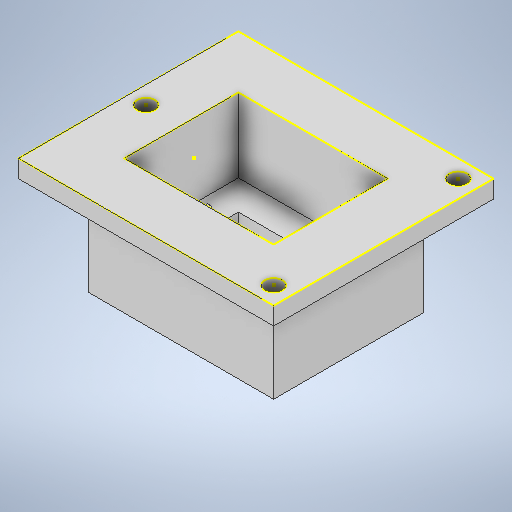
# Autodesk Inventor part: servo_holder_V2
Saved by Autodesk Inventor 2025.3 (Build 293356000, 356)
## iProperties
Created: 2026-04-11
Part Number: servo_holder_V2
Material: Generic
Document SubType Name: Modeling
Designer: kamal
Density: 1 g/cm^3
Appearance: Default
Author: kamal
## iProperties of the stored document servo_holder_V2_3DPrint.ipt
Created: 2026-04-12
Part Number: servo_holder_V2_3DPrint
Material: Generic
Document SubType Name: Modeling
Designer: kamal
Density: 1 g/cm^3
Appearance: Default
Author: kamal
Autodesk Inventor part; units mm, degrees
ref_plane "YZ Plane" through (0, 0, 0) normal (1, 0, 0) x (0, 1, 0)
ref_plane "XZ Plane" through (0, 0, 0) normal (0, 1, 0) x (-1, 0, 0)
sketch "Sketch1" plane through (0, 0, 0) normal (0, 0, 1) x (1, 0, 0)
  line L0 (0, 0) -> (22.6, 0)
  line L1 (22.6, 0) -> (22.6, 12.6)
  line L2 (22.6, 12.6) -> (0, 12.6)
  line L3 (0, 12.6) -> (0, 0)
  line L4 (-4.9, 17.5) -> (27.5, 17.5)
  line L5 (27.5, 17.5) -> (27.5, -4.9)
  line L6 (27.5, -4.9) -> (-4.9, -4.9)
  line L7 (-4.9, -4.9) -> (-4.9, 17.5)
  dimension "d0" = 22.6
  dimension "d1" = 12.6
  dimension "d2" = 4.9
  constraints: 16 end point, 4 parallel, 2 perpendicular, 1 horizontal, 3 other
  measures "d0" distance of L2.end L1.end
  measures "d1" distance of L1.end L0.end
  measures "d2" distance between parallel lines of L2 L4
extrude "Extrusion1" add sketch "Sketch1" along normal blind 17
sketch "Sketch2" plane through (0, 0, 0) normal (0, 0, -1) x (-1, 0, 0)
  line L0 (4.9, -4.9) -> (-27.5, -4.9) projected
  line L1 (-27.5, -4.9) -> (-27.5, 17.5) projected
  line L2 (-27.5, 17.5) -> (4.9, 17.5) projected
  line L3 (4.9, 17.5) -> (4.9, -4.9) projected
  point P0 (0, 0)
extrude "Extrusion2" add sketch "Sketch2" along normal blind 5
sketch "Sketch3" plane through (0, 0, 17) normal (0, 0, 1) x (1, 0, 0)
  line L0 (-4.9, -4.9) -> (27.5, -4.9) projected
  line L1 (27.5, -4.9) -> (27.5, 17.5) projected
  line L2 (27.5, 17.5) -> (-4.9, 17.5) projected
  line L3 (-4.9, 17.5) -> (-4.9, -4.9) projected
  line L4 (0, 0) -> (0, 12.6) projected
  line L5 (0, 12.6) -> (22.6, 12.6) projected
  line L6 (22.6, 12.6) -> (22.6, 0) projected
  line L7 (22.6, 0) -> (0, 0) projected
  line L8 (-9.9, -9.9) -> (32.5, -9.9)
  line L9 (32.5, -9.9) -> (32.5, 22.5)
  line L10 (32.5, 22.5) -> (-9.9, 22.5)
  line L11 (-9.9, 22.5) -> (-9.9, -9.9)
  line L12 (-4.9, 6.3) -> (-2.6, 6.3) construction
  line L13 (27.5, 17.5) -> (27.5, -4.9) projected
  line L14 (27.5, 6.3) -> (25.2, 6.3) construction
  circle A0 centre (-2.6, 6.3) radius 1
  circle A1 centre (25.2, 6.3) radius 1
  dimension "d7" = 5
  dimension "d10" = 2.3
  dimension "d11" = 2.3
  dimension "d12" = 2
  dimension "d13" = 2
  constraints: 12 end point, 2 centre point, 2 coincident, 2 horizontal, 2 midpoint, 3 other
  measures "d7" distance between parallel lines of L3 L11
  measures "d10" distance of L12.start L12.end
  measures "d11" distance of L14.start L14.end
  measures "d12" diameter of A0
  measures "d13" diameter of A1
extrude "Extrusion4" add sketch "Sketch3" along normal blind 5 contours A0 | A1
chamfer "Chamfer1" distance 0.5 angle 45 2 edges at (-3.6, 6.3, 22) (24.2, 6.3, 22)
ref_plane "Work Plane1" through (0, 0, 12) normal (0, 0, 1) x (1, 0, 0)
sketch "Sketch5" plane through (0, 0, 12) normal (0, 0, 1) x (1, 0, 0)
  line L0 (-4.9, -4.9) -> (27.5, -4.9) projected
  line L1 (27.5, -4.9) -> (27.5, 17.5) projected
  line L2 (27.5, 17.5) -> (-4.9, 17.5) projected
  line L3 (-4.9, 17.5) -> (-4.9, -4.9) projected
  line L4 (32.5, -9.9) -> (-9.9, -9.9)
  line L5 (-9.9, -9.9) -> (-9.9, 22.5)
  line L6 (-9.9, 22.5) -> (32.5, 22.5)
  line L7 (32.5, 22.5) -> (32.5, -9.9)
  point P0 (0, 0)
  dimension "d21" = 5
  constraints: 8 end point, 3 other
  measures "d21" distance between parallel lines of L0 L4
extrude "Extrusion5" add sketch "Sketch5" along normal blind 5
sketch "Sketch14" plane through (0, 0, 17) normal (0, 0, 1) x (1, 0, 0)
  line L0 (22.6, 12.6) -> (22.6, 0) projected
  line L1 (0, 12.6) -> (22.6, 12.6) projected
  line L2 (0, 0) -> (0, 12.6) projected
  line L3 (22.6, 0) -> (0, 0) projected
  line L4 (-9.9, -9.9) -> (-9.9, 22.5)
  line L5 (-9.9, 22.5) -> (32.5, 22.5)
  line L6 (32.5, 22.5) -> (32.5, -9.9)
  line L7 (32.5, -9.9) -> (-9.9, -9.9)
  line L8 (-14.9, -14.9) -> (-14.9, 27.5)
  line L9 (-14.9, 27.5) -> (37.5, 27.5)
  line L10 (37.5, 27.5) -> (37.5, -14.9)
  line L11 (37.5, -14.9) -> (-14.9, -14.9)
  dimension "d52" = 9.9
  dimension "d53" = 5
  constraints: 16 end point, 6 other
  measures "d52" distance between parallel lines of L3 L7
  measures "d53" distance between parallel lines of L7 L11
extrude "Extrusion11" add sketch "Sketch14" along normal blind 16 contours L8 L9 L10 L11
sketch "Sketch15" plane through (0, 0, 33) normal (0, 0, 1) x (1, 0, 0)
  line L0 (-14.9, 27.5) -> (-14.9, -14.9) projected
  line L1 (-14.9, -14.9) -> (37.5, -14.9) projected
  line L2 (37.5, -14.9) -> (37.5, 27.5) projected
  line L3 (37.5, 27.5) -> (-14.9, 27.5) projected
  line L4 (47.5, -24.9) -> (-24.9, -24.9)
  line L5 (-24.9, -24.9) -> (-24.9, 37.5)
  line L6 (-24.9, 37.5) -> (47.5, 37.5)
  line L7 (47.5, 37.5) -> (47.5, -24.9)
  line L8 (32.5, -9.9) -> (-9.9, -9.9) projected
  line L9 (-9.9, -9.9) -> (-9.9, 22.5) projected
  line L10 (-9.9, 22.5) -> (32.5, 22.5) projected
  line L11 (32.5, 22.5) -> (32.5, -9.9) projected
  point P0 (0, 0)
  dimension "d56" = 10
  constraints: 8 end point, 3 other
  measures "d56" distance between parallel lines of L1 L4
extrude "Extrusion12" add sketch "Sketch15" along normal blind 5 contours L3 L2 L1 L0 | L4 L5 L6 L7
sketch "Sketch16" plane through (0, 0, 33) normal (0, 0, -1) x (-1, 0, 0)
  line L0 (-37.5, -14.9) -> (-37.5, 27.5) projected
  line L1 (14.9, -14.9) -> (-37.5, -14.9) projected
  line L2 (14.9, 27.5) -> (14.9, -14.9) projected
  line L3 (-37.5, 27.5) -> (14.9, 27.5) projected
  line L4 (9.9, 22.5) -> (9.9, -9.9) projected
  line L5 (9.9, -9.9) -> (-32.5, -9.9) projected
  line L6 (-32.5, -9.9) -> (-32.5, 22.5) projected
  line L7 (-32.5, 22.5) -> (9.9, 22.5) projected
  line L8 (-42.5, 32.5) -> (-42.5, -19.9) construction
  line L9 (-42.5, -19.9) -> (19.9, -19.9) construction
  line L10 (19.9, -19.9) -> (19.9, 32.5) construction
  line L11 (19.9, 32.5) -> (-42.5, 32.5) construction
  circle A0 centre (19.9, 6.3) radius 2.5
  circle A1 centre (-42.5, 32.5) radius 2.5
  circle A2 centre (-42.5, -19.9) radius 2.5
  point P0 (0, 0)
  dimension "d59" = 5
  dimension "d60" = 5
  dimension "d61" = 5
  dimension "d62" = 5
  constraints: 8 end point, 3 centre point, 2 coincident, 1 midpoint, 3 other
  measures "d59" distance between parallel lines of L0 L8
  measures "d60" diameter of A0
  measures "d61" diameter of A1
  measures "d62" diameter of A2
extrude "Extrusion13" cut sketch "Sketch16" against normal blind 5 contours A0 | A1 | A2
sketch "Sketch17" plane through (-4.9, -4.9, -5) normal (-1, 0, 0) x (0, 0, 1)
  line L0 (-10, 15.2) -> (10, 15.2)
  line L1 (10, 15.2) -> (10, 7.2)
  line L2 (10, 7.2) -> (-10, 7.2)
  line L3 (-10, 7.2) -> (-10, 15.2)
  line L4 (0, 22.4) -> (0, 0) projected
  line L5 (-10, 15.2) -> (10, 7.2) construction
  line L6 (10, 15.2) -> (-10, 7.2) construction
  line L7 (5, 15.2) -> (5, 7.2)
  line L8 (0, 11.2) -> (5, 11.2)
  point P0 (5, 4.9)
  dimension "d65" = 20
  dimension "d66" = 8
  dimension "d67" = 5
  constraints: 16 end point, 4 midpoint, 2 parallel, 2 perpendicular, 2 point on line, 1 horizontal
  measures "d65" distance of L1.end L2.end
  measures "d66" distance of L0.end L1.end
  measures "d67" distance of L8.start L8.end
extrude "Extrusion14" cut sketch "Sketch17" against normal blind 5 contours L0 L1 L2 L7
sketch "Sketch18" plane through (0, 0, 12) normal (0, 0, -1) x (-1, 0, 0)
  line L0 (-32.5, 22.5) -> (9.9, 22.5) projected
  line L1 (-32.5, -9.9) -> (-32.5, 22.5) projected
  line L2 (9.9, -9.9) -> (-32.5, -9.9) projected
  line L3 (9.9, 22.5) -> (9.9, -9.9) projected
  line L4 (4.9, -4.9) -> (4.9, 17.5) projected
  line L5 (-27.5, -4.9) -> (4.9, -4.9) projected
  line L6 (-27.5, 17.5) -> (-27.5, -4.9) projected
  line L7 (4.9, 17.5) -> (-27.5, 17.5) projected
  point P0 (0, 0)
extrude "Extrusion15" add sketch "Sketch18" along normal blind 7
sketch "Sketch20" plane through (-4.9, -4.9, -5) normal (-1, 0, 0) x (0, 0, 1)
  line L0 (5, 7.2) -> (0, 7.2)
  line L1 (5, 15.2) -> (10, 15.2) projected
  line L2 (5, 15.2) -> (0, 15.2)
  line L3 (0, 15.2) -> (0, 7.2)
  line L4 (5, 15.2) -> (5, 17.5) projected
  line L5 (5, 7.2) -> (5, 15.2)
  point P0 (5, 4.9)
  dimension "d74" = 10
  constraints: 8 end point, 2 horizontal, 1 collinear, 1 perpendicular
  measures "d74" distance from line of L1.end L3
extrude "Extrusion17" cut sketch "Sketch20" against normal blind 12
sketch "Sketch21" plane through (0, 0, 17) normal (0, 0, -1) x (-1, 0, 0)
  line L0 (-32.5, -9.9) -> (9.9, -9.9) projected
  line L1 (9.9, -9.9) -> (9.9, 22.5) projected
  line L2 (9.9, 22.5) -> (-32.5, 22.5) projected
  line L3 (-32.5, 22.5) -> (-32.5, -9.9) projected
  line L4 (0, 2.3) -> (0, 10.3) projected
  line L5 (4.9, 2.3) -> (0, 2.3) projected
  line L6 (4.9, -4.9) -> (4.9, 2.3) projected
  line L7 (-27.5, -4.9) -> (4.9, -4.9) projected
  line L8 (-27.5, 17.5) -> (-27.5, -4.9) projected
  line L9 (4.9, 17.5) -> (-27.5, 17.5) projected
  line L10 (4.9, 10.3) -> (4.9, 17.5) projected
  line L11 (4.9, 10.3) -> (0, 10.3) projected
  line L12 (-37.5, -14.9) -> (-37.5, 27.5) projected
  line L13 (14.9, -14.9) -> (-37.5, -14.9) projected
  line L14 (14.9, 27.5) -> (14.9, -14.9) projected
  line L15 (-37.5, 27.5) -> (14.9, 27.5) projected
  line L16 (9.9, 22.5) -> (9.9, -9.9) projected
  line L17 (9.9, -9.9) -> (-32.5, -9.9) projected
  line L18 (-32.5, -9.9) -> (-32.5, 22.5) projected
  line L19 (-32.5, 22.5) -> (9.9, 22.5) projected
  point P0 (0, 0)
extrude "Extrusion18" add sketch "Sketch21" along normal blind 12 contours L12 L15 L14 L13
sketch "Sketch22" plane through (0, 0, 17) normal (0, 0, 1) x (1, 0, 0)
  line L0 (0, 12.6) -> (22.6, 12.6) projected
  line L1 (22.6, 12.6) -> (22.6, 0) projected
  line L2 (22.6, 0) -> (0, 0) projected
  line L3 (0, 0) -> (0, 12.6) projected
  line L4 (24.1, 14.1) -> (-1.5, 14.1)
  line L5 (-1.5, 14.1) -> (-1.5, -1.5)
  line L6 (-1.5, -1.5) -> (24.1, -1.5)
  line L7 (24.1, -1.5) -> (24.1, 14.1)
  dimension "d79" = 1.5
  constraints: 8 end point, 3 other
  measures "d79" distance between parallel lines of L0 L4
extrude "Extrusion19" cut sketch "Sketch22" against normal blind 17
sketch "Sketch23" plane through (0, 0, 38) normal (0, 0, 1) x (1, 0, 0)
  circle A0 centre (-19.9, 6.3) radius 2.5 projected
  circle A1 centre (42.5, 32.5) radius 2.5 projected
  circle A2 centre (42.5, -19.9) radius 2.5 projected
  line L0 (47.5, 37.5) -> (-24.9, 37.5) projected
  line L1 (-24.9, 37.5) -> (-24.9, -24.9) projected
  line L2 (-24.9, -24.9) -> (47.5, -24.9) projected
  line L3 (47.5, -24.9) -> (47.5, 37.5) projected
  line L4 (32.5, -9.9) -> (-9.9, -9.9) projected
  line L5 (-9.9, -9.9) -> (-9.9, 22.5) projected
  line L6 (-9.9, 22.5) -> (32.5, 22.5) projected
  line L7 (32.5, 22.5) -> (32.5, -9.9) projected
  point P0 (0, 0)
equation "\"d63\" = d62"
equation "\"d68\" = d62"
body "Solid1"
